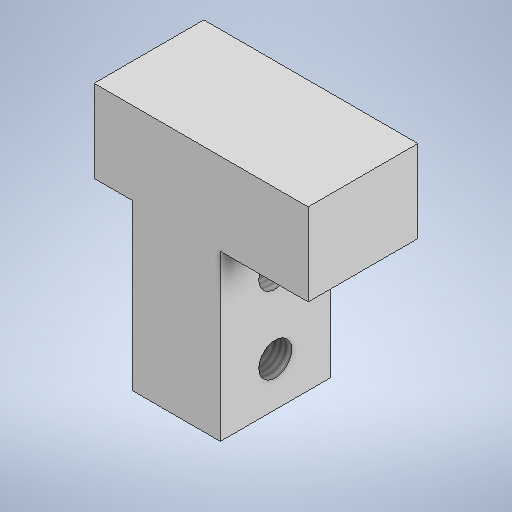
# Autodesk Inventor part: Connector2
Saved by Autodesk Inventor 2025 (Build 290162000, 162)
## iProperties
Created: 2024-09-26
Part Number: Connector2
Material: Generic
Document SubType Name: Modeling
Designer: DMIADX
Density: 1 g/cm^3
Appearance: Default
Author: DMIADX
Autodesk Inventor part; units mm, degrees
ref_plane "YZ Plane" through (0, 0, 0) normal (1, 0, 0) x (0, 1, 0)
ref_plane "XZ Plane" through (0, 0, 0) normal (0, 1, 0) x (-1, 0, 0)
ref_plane "XY Plane" through (0, 0, 0) normal (0, 0, 1) x (1, 0, 0)
sketch "Sketch1" plane through (0, 0, 0) normal (0, 0, 1) x (1, 0, 0)
  line L0 (0, 0) -> (-8, 0)
  line L1 (-8, 0) -> (-8, 15)
  line L2 (-8, 15) -> (0, 15)
  line L3 (0, 15) -> (0, 0)
  line L4 (8, 22.5) -> (-11.5, 22.5)
  line L5 (-11.5, 22.5) -> (-11.5, 15)
  line L6 (-11.5, 15) -> (8, 15)
  line L7 (8, 15) -> (8, 22.5)
  line L8 (0, 15) -> (1, 15)
  line L9 (0, 14) -> (0, 15)
  point P0 (0.5, 15)
  point P1 (0.5, 14)
  dimension "d0" = 15
  dimension "d1" = 1
  dimension "d3" = 19.5
  dimension "d4" = 3.5
  dimension "d5" = 8
  dimension "d6" = 7.5
  constraints: 20 end point, 4 parallel, 3 horizontal, 2 perpendicular, 1 midpoint, 1 point on line
  measures "d0" distance between parallel lines of L0 L2
  measures "d1" distance of point (0.5, 15) point (0.5, 14)
  measures "d3" distance between parallel lines of L7 L5
  measures "d4" distance between parallel lines of L5 L1
  measures "d5" distance between parallel lines of L3 L1
  measures "d6" distance of L4.end L5.end
extrude "Extrusion1" add sketch "Sketch1" along normal mid plane 10
sketch "Sketch2" plane through (0, 0, 5) normal (1, 0, 0) x (0, 0, -1)
  circle A0 centre (5, 4) radius 1.5
  circle A1 centre (5, 11) radius 1.5
  line L0 (10, 14) -> (0, 14) projected
  line L1 (10, 0) -> (0, 0) projected
  line L2 (10, 15) -> (0, 15) projected
  point P0 (5, 0)
  point P1 (5, 0)
  point P2 (5, 0)
  dimension "d9" = 3
  dimension "d10" = 3
  dimension "d12" = 7
  dimension "d19" = 4
  constraints: 2 centre point, 2 midpoint, 2 vertical alignment
  measures "d9" diameter of A0
  measures "d10" diameter of A1
  measures "d12" distance of A1.centre A0.centre
  measures "d19" distance from line of A1.centre L2
extrude "Extrusion2" cut sketch "Sketch2" against normal through all
thread "Thread1" size "M3x0.5" class "6H" standard "ANSI Metric M Profile" full length
thread "Thread2" size "M3x0.5" class "6H" standard "ANSI Metric M Profile" full length
body "Solid1"
